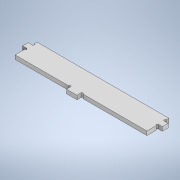
# Autodesk Inventor part: Level 1 Support Mid
Saved by Autodesk Inventor 2020 (Build 240168000, 168)
## iProperties
Created: 2020-03-07
Part Number: Level 1 Support Mid
Material: Wood (Maple)
Document SubType Name: Modeling
Designer: Daniel Wikman
Density: 0.67 g/cm^3
Appearance: Default
Author: Daniel Wikman
Autodesk Inventor part; units mm, degrees
ref_plane "YZ Plane" through (0, 0, 0) normal (1, 0, 0) x (0, 1, 0)
ref_plane "XZ Plane" through (0, 0, 0) normal (0, 1, 0) x (-1, 0, 0)
ref_plane "XY Plane" through (0, 0, 0) normal (0, 0, 1) x (1, 0, 0)
sketch "Sketch1" plane through (0, 0, 0) normal (0, 1, 0) x (-1, 0, 0)
  arc A0 (54.4292, -38.5976) -> (54.4292, -42.0976) centre (54.4292, -40.3476) ccw
  arc A1 (54.4292, -25.0976) -> (54.4292, -28.5976) centre (54.4292, -26.8476) ccw
  line L0 (61.4292, -38.5976) -> (61.4292, -28.5976)
  line L1 (-42.6541, -8.5976) -> (-42.6541, -1.5976)
  line L2 (61.4292, -28.5976) -> (54.4292, -28.5976)
  line L3 (61.4292, -38.5976) -> (54.4292, -38.5976)
  line L4 (54.4292, -25.0976) -> (54.4292, -8.5976)
  line L5 (54.4292, -42.0976) -> (54.4292, -47.0976)
  line L6 (-60.9041, -44.0976) -> (-60.9041, -33.5976)
  arc A2 (-176.2375, -42.0976) -> (-176.2375, -38.5976) centre (-176.2375, -40.3476) ccw
  arc A3 (-176.2375, -28.5976) -> (-176.2375, -25.0976) centre (-176.2375, -26.8476) ccw
  line L7 (-183.2375, -38.5976) -> (-183.2375, -28.5976)
  line L8 (-183.2375, -28.5976) -> (-176.2375, -28.5976)
  line L9 (-183.2375, -38.5976) -> (-176.2375, -38.5976)
  line L10 (-176.2375, -25.0976) -> (-176.2375, -8.5976)
  line L11 (-176.2375, -42.0976) -> (-176.2375, -47.0976)
  line L12 (54.4292, -47.0976) -> (-176.2375, -47.0976)
  arc A4 (-42.6541, -8.5976) -> (-39.1541, -8.5976) centre (-40.9041, -8.5976) ccw
  line L13 (-39.1541, -8.5976) -> (54.4292, -8.5976)
  line L14 (-60.9041, -1.5976) -> (-60.9041, -8.5976)
  arc A5 (-64.4041, -8.5976) -> (-60.9041, -8.5976) centre (-62.6541, -8.5976) ccw
  line L15 (-64.4041, -8.5976) -> (-176.2375, -8.5976)
  line L16 (-42.6541, -1.5976) -> (-60.9041, -1.5976)
  point P0 (0, 0)
  dimension "d2" = 3.5
  dimension "d5" = 3.5
  dimension "d9" = 7
  dimension "d11" = 10
  dimension "d32" = 5
  dimension "d33" = 230.6667
  dimension "d36" = 7
  dimension "d42" = 3.5
  dimension "d43" = 97.0833
  dimension "d44" = 3.5
  dimension "d45" = 18.25
  dimension "d46" = 20
  constraints: 34 end point, 12 point on circle, 9 symmetric about line, 6 centre point, 6 vertical, 4 horizontal, 2 tangent, 1 parallel, 1 perpendicular, 3 other
  measures "d2" diameter of A0
  measures "d5" diameter of A1
  measures "d9" distance of L2.end L0.end
  measures "d11" distance of L0.start L0.end
  measures "d32" distance of L5.start L5.end
  measures "d33" distance of L5.end L11.end
  measures "d36" distance between parallel lines of L0 L4
  measures "d42" diameter of A4
  measures "d43" distance between parallel lines of L4 L1
  measures "d44" diameter of A5
  measures "d45" distance between parallel lines of L1 L14
  measures "d46" distance between parallel lines of L2 L13
extrude "Extrusion1" add sketch "Sketch1" along normal blind 7
body "Solid1"
